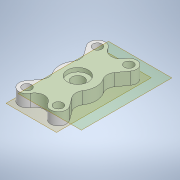
# Autodesk Inventor part: shaft encap lid
Saved by Autodesk Inventor 2022 (Build 260153000, 153)
## iProperties
Created: 2022-11-12
Part Number: shaft encap lid
Material: Generic
Document SubType Name: Modeling
Designer: efred
Density: 1 g/cm^3
Appearance: Default
Author: efred
Autodesk Inventor part; units mm, degrees
ref_plane "YZ Plane" through (0, 0, 0) normal (1, 0, 0) x (0, 1, 0)
ref_plane "XZ Plane" through (0, 0, 0) normal (0, 1, 0) x (-1, 0, 0)
ref_plane "XY Plane" through (0, 0, 0) normal (0, 0, 1) x (1, 0, 0)
ref_plane "Work Plane1" through (9.1457, 10.0679, 19.8187) normal (0, 1, 0) x (-1, 0, 0)
sketch "Sketch1" plane through (9.1457, 10.0679, 19.8187) normal (0, 1, 0) x (-1, 0, 0)
  circle A0 centre (-8, -17.9) radius 2 construction
  circle A1 centre (-8, 17.9) radius 2 construction
  arc A2 (7.7389, -5.1575) -> (7.7389, 5.1575) centre (0, 0) ccw projected
  arc A3 (-4.4444, 19.7325) -> (-11.2421, 15.5572) centre (-8, 17.9) ccw projected
  line L0 (-7.847, 10.8589) -> (-11.2421, 15.5572) projected
  arc A4 (-7.7389, 5.1575) -> (-7.847, 10.8589) centre (-11.8996, 7.9303) ccw projected
  arc A5 (-7.847, -10.8589) -> (-7.7389, -5.1575) centre (-11.8996, -7.9303) ccw projected
  line L1 (-11.2421, -15.5572) -> (-7.847, -10.8589) projected
  arc A6 (-11.2421, -15.5572) -> (-4.4444, -19.7325) centre (-8, -17.9) ccw projected
  circle A7 centre (0, 0) radius 7.3 construction
  circle A8 centre (0, 0) radius 5 construction
  circle A9 centre (0, 0) radius 2.5 construction
  circle A10 centre (-8, 17.9) radius 2.3
  circle A11 centre (-8, -17.9) radius 2.3
  circle A12 centre (8, -17.9) radius 2 construction
  circle A13 centre (8, 17.9) radius 2 construction
  arc A14 (4.4444, -19.7325) -> (-4.4444, -19.7325) centre (0, -22.0231) ccw projected
  arc A15 (4.4444, -19.7325) -> (11.2421, -15.5572) centre (8, -17.9) ccw projected
  line L2 (11.2421, -15.5572) -> (7.847, -10.8589) projected
  arc A16 (7.7389, -5.1575) -> (7.847, -10.8589) centre (11.8996, -7.9303) ccw projected
  arc A17 (7.847, 10.8589) -> (7.7389, 5.1575) centre (11.8996, 7.9303) ccw projected
  line L3 (7.847, 10.8589) -> (11.2421, 15.5572) projected
  arc A18 (11.2421, 15.5572) -> (4.4444, 19.7325) centre (8, 17.9) ccw projected
  arc A19 (-4.4444, 19.7325) -> (4.4444, 19.7325) centre (0, 22.0231) ccw projected
  circle A20 centre (8, -17.9) radius 2.3
  circle A21 centre (8, 17.9) radius 2.3
  arc A22 (1.8, 2.1448) -> (-1.8, 2.1448) centre (0, 0) ccw construction
  line L4 (-1.8, -2.1448) -> (-1.8, 2.1448) construction
  arc A23 (-1.8, -2.1448) -> (1.8, -2.1448) centre (0, 0) ccw construction
  line L5 (1.8, 2.1448) -> (1.8, -2.1448) construction
  line L6 (1.5, 2) -> (1.5, -2) projected
  arc A24 (-1.5, -2) -> (1.5, -2) centre (0, 0) ccw projected
  line L7 (-1.5, -2) -> (-1.5, 2) projected
  arc A25 (1.5, 2) -> (-1.5, 2) centre (0, 0) ccw projected
  circle A26 centre (0, 0) radius 2.8
  arc A27 (-7.7389, 5.1575) -> (-7.7389, -5.1575) centre (0, 0) ccw projected
  point P0 (9.1457, -19.8187)
  point P1 (-13.1394, 9.646)
  point P2 (-13.1394, -9.646)
  point P3 (13.1394, -9.646)
  point P4 (13.1394, 9.646)
  point P5 (-11.8996, 7.9303)
  point P6 (-11.8996, -7.9303)
  point P7 (11.8996, -7.9303)
  point P8 (11.8996, 7.9303)
  point P9 (11.8996, -7.9303)
  point P10 (11.8996, 7.9303)
  point P11 (-11.8996, 7.9303)
  point P12 (-11.8996, -7.9303)
  point P13 (11.8996, -7.9303)
  point P14 (11.8996, 7.9303)
  point P15 (0, 0)
  point P16 (11.8996, -7.9303)
  point P17 (11.8996, 7.9303)
  point P18 (11.8996, -7.9303)
  point P19 (11.8996, 7.9303)
  dimension "d1" = 0.3
  dimension "d2" = 0.3
  dimension "d8" = 0.3
  dimension "d9" = 0.3
  dimension "d20" = 0.3
  constraints: 5 centre point
  measures "d1" radial gap between concentric circles of A1 A10
  measures "d2" radial gap between concentric circles of A0 A11
  measures "d8" radial gap between concentric circles of A12 A20
  measures "d9" radial gap between concentric circles of A13 A21
  measures "d20" radial gap between concentric circles of A9 A26
ref_plane "Work Plane2" through (17.1457, 15.7679, 19.8187) normal (0, -1, 0) x (-1, 0, 0)
extrude "Extrusion1" add sketch "Sketch1" along normal up to surface (5.7 mm away) contours A16 L2 A15 A14 A6 L1 A5 A27 A4 L0 A3 A19 A18 L3 A17 A2
sketch "Sketch3" plane through (9.1457, 15.7679, 41.8418) normal (0, 1, 0) x (1, 0, 0)
  circle A0 centre (0, 22.0231) radius 5 construction
  circle A1 centre (0, 22.0231) radius 5.3
  point P0 (-9.1457, 41.8418)
  dimension "d11" = 0.3
  constraints: 1 centre point
  measures "d11" radial gap between concentric circles of A0 A1
ref_plane "Work Plane4" through (9.1457, 13.7679, 19.8187) normal (0, -1, 0) x (-1, 0, 0)
extrude "Extrusion3" cut sketch "Sketch3" against normal up to surface (2 mm away)
sketch "Sketch4" plane through (9.1457, 13.7679, 19.8187) normal (0, 1, 0) x (1, 0, 0)
  circle A0 centre (0, 0) radius 3.8 projected
  circle A1 centre (0, 0) radius 5.3 projected
  point P0 (-9.1457, 19.8187)
extrude "Extrusion4" cut sketch "Sketch4" against normal blind 0.1
ref_plane "Work Plane5" through (1.2414, 11.6271, 11.9106) normal (0, 1, 0) x (0, 0, 1)
body "Solid1"
